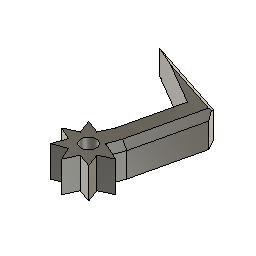
claw_part_right_Asheeyana_Ahmed (Autodesk Fusion 360 design; units mm, degrees)
Autodesk Fusion 360 part; units mm, degrees
sketch "Sketch1" plane through (0, 0, 0) normal (0, 0, 1) x (1, 0, 0)
  line L0 (29.7102, -20.9929) -> (0, -20.9929)
  line L1 (-7, 31.5) -> (20.239, 31.5)
  line L2 (20.239, 31.5) -> (29.7102, -20.9929)
  line L3 (-7, 31.5) -> (0, -20.9929)
  line L4 (3.9378, -2.5628) -> (1.375, -8.75)
  line L5 (1.375, -8.75) -> (3.9378, -14.9372)
  line L6 (3.9378, -14.9372) -> (10.125, -17.5)
  line L7 (10.125, -17.5) -> (16.3122, -14.9372)
  line L8 (16.3122, -14.9372) -> (18.875, -8.75)
  line L9 (18.875, -8.75) -> (16.3122, -2.5628)
  line L10 (16.3122, -2.5628) -> (10.125, 0)
  line L11 (15.1989, 4.3652) -> (15.1875, 4.3554)
  line L12 (-7, 31.5) -> (14.4889, 18.96)
  line L13 (-7, 31.5) -> (21.9586, 21.9692)
  line L14 (21.9586, 21.9692) -> (16.3122, -2.5628)
  line L15 (10.125, 0) -> (13.5018, 14.6711)
  line L16 (10.125, 0) -> (3.9378, -2.5628)
  circle A0 centre (10.125, -8.75) radius 2.5
  circle A1 centre (10.125, -8.75) radius 5
  line L17 (7.0314, -1.2814) -> (10.125, -8.75) construction
  line L18 (10.125, 0) -> (8.2116, -4.1306)
  line L19 (8.2116, -4.1306) -> (3.9378, -2.5628)
  line L20 (3.9378, -2.5628) -> (5.5056, -6.8366)
  line L21 (5.5056, -6.8366) -> (1.375, -8.75)
  line L22 (1.375, -8.75) -> (5.5056, -10.6634)
  line L23 (5.5056, -10.6634) -> (3.9378, -14.9372)
  line L24 (3.9378, -14.9372) -> (8.2116, -13.3694)
  line L25 (8.2116, -13.3694) -> (10.125, -17.5)
  line L26 (10.125, -17.5) -> (12.0384, -13.3694)
  line L27 (12.0384, -13.3694) -> (16.3122, -14.9372)
  line L28 (16.3122, -14.9372) -> (14.7444, -10.6634)
  line L29 (14.7444, -10.6634) -> (18.875, -8.75)
  line L30 (18.875, -8.75) -> (14.7444, -6.8366)
  line L31 (14.7444, -6.8366) -> (16.3122, -2.5628)
  line L32 (16.3122, -2.5628) -> (12.0384, -4.1306)
  line L33 (12.0384, -4.1306) -> (10.125, 0)
  line L34 (13.5018, 14.6711) -> (14.4889, 18.96)
  point P0 (10.125, -8.75)
  dimension "d3" = 5
  dimension "d4" = 10
  dimension "d6" = 360
  constraint horizontal L0
  constraint parallel L0 L1
  constraint coincident L2 L13.end
  constraint parallel L14 L15
  constraint coincident L15 L12.end
  constraint coincident P0 A0.centre
  constraint concentric A0 A1
  constraint midpoint L16 L17.start
  constraint coincident A1 L18.end
  constraint coincident L17 L18.end
  measures "d3" diameter of A0
  measures "d4" diameter of A1
extrude "Extrude1" add sketch "Sketch1" along normal blind 10 contours L10 L12 L13 L14 L15 L34 | L10 L32 L33 | A1 L31 L32 | A1 L29 L30 | A1 L18 L33 | A1 | A1 L27 L28 | A1 L19 L20 | A1 L25 L26 | A1 L21 L22 | A1 L23 L24
chamfer "Chamfer1" distance 3 angle 45 1 edges at (21.9586, 21.9692, 5)
chamfer "Chamfer2" distance 2 angle 45 1 edges at (6.0545, 27.2035, 10)
chamfer "Chamfer3" distance 2 angle 45 2 edges at (15.5283, -4.6997, 10) (18.7989, 8.2414, 10)
